Autodesk Inventor part; units mm, degrees
(part 4 of 4)
sketch "Эскиз10" plane through (23.5, 10.85, -93.6349) normal (0, 0, 1) x (1, 0, 0)
  arc A0 (0, 0) -> (-2.0546, 2.8471) centre (-3, 0) ccw projected
  line L0 (-2.0546, -10.85) -> (-2.0546, 2.8471) construction
  line L1 (0, -10.85) -> (-2.0546, -10.85) construction
  line L2 (0, -10.85) -> (0, 0) construction
  spline S0 degree 4 poles (-4.4081, 2.9941) (-4.3815, 2.997) (-4.3546, 2.999) (-4.3274, 3) (-4.3, 3) knots 0 0 0 0 0 1 1 1 1 1 projected
  line L3 (-4.4081, -1.0919) -> (-4.4081, 2.9941) construction
  line L4 (-3.5, -2) -> (-4.4081, -1.0919) projected
  line L5 (-3.5, -7) -> (-3.5, -2) construction
  line L6 (-4.4081, -7) -> (-3.5, -7) construction
  line L7 (-4.4081, -10.85) -> (-4.4081, -7) construction
  line L8 (-2.0546, -10.85) -> (-4.4081, -10.85) construction
  line L9 (-2.0546, -10.85) -> (-2.0546, 2.8471) construction
  spline S1 degree 6 poles (-3, 3) (-2.9139, 3) (-2.8267, 2.997) (-2.7386, 2.991) (-2.6499, 2.9817) (-2.5611, 2.9691) (-2.4019, 2.9407) (-2.3314, 2.926) (-2.2612, 2.9092) (-2.1915, 2.8904) (-2.1226, 2.8697) (-2.0546, 2.8471) knots 0 0 0 0 0 0 0 0.556009 0.556009 0.556009 0.556009 0.556009 1 1 1 1 1 1 1 projected
  line L10 (-4.3, 3) -> (-3, 3) projected
  arc A1 (-4.4081, 2.9941) -> (-5.3, 2) centre (-4.3, 2) ccw projected
  line L11 (-5.3, -0.2) -> (-5.3, 2) projected
  line L12 (-4.4081, -1.0919) -> (-5.3, -0.2) projected
  line L13 (-4.4081, -1.0919) -> (-4.4081, 2.9941) construction
  line L14 (-42.5919, -1.0919) -> (-42.5919, 2.9941) projected
  arc A2 (-41.7, 2) -> (-42.5919, 2.9941) centre (-42.7, 2) ccw projected
  line L15 (-42.5919, -1.0919) -> (-42.5919, 2.9941) projected
  line L16 (-41.7, -0.2) -> (-42.5919, -1.0919) projected
  line L17 (-41.7, -0.2) -> (-41.7, 2) projected
  spline S2 degree 7 poles (-42.7, 3) (-42.6843, 3) (-42.6687, 2.9997) (-42.6532, 2.9991) (-42.6378, 2.9983) (-42.6224, 2.9972) (-42.6071, 2.9958) (-42.5919, 2.9941) knots 0 0 0 0 0 0 0 0 1 1 1 1 1 1 1 1 projected
  line L18 (-44, 3) -> (-42.7, 3) projected
  spline S3 degree 5 poles (-44.9454, 2.8471) (-44.8643, 2.8741) (-44.782, 2.8982) (-44.6986, 2.9194) (-44.6145, 2.9376) (-44.4235, 2.9719) (-44.3163, 2.9862) (-44.2095, 2.9955) (-44.1039, 3) (-44, 3) knots 0 0 0 0 0 0 0.440959 0.440959 0.440959 0.440959 1 1 1 1 1 1 projected
  line L19 (-44.9454, -10.85) -> (-44.9454, 2.8471) construction
  line L20 (-42.5919, -10.85) -> (-44.9454, -10.85) construction
  line L21 (-42.5919, -10.85) -> (-42.5919, -7) construction
  line L22 (-43.5, -7) -> (-42.5919, -7) construction
  line L23 (-43.5, -7) -> (-43.5, -2) construction
  line L24 (-42.5919, -1.0919) -> (-43.5, -2) projected
  line L25 (-42.5919, -1.0919) -> (-42.5919, 2.9941) projected
  arc A3 (-44.9454, 2.8471) -> (-47, 0) centre (-44, 0) ccw projected
  line L26 (-47, -10.85) -> (-47, 0) construction
  line L27 (-44.9454, -10.85) -> (-47, -10.85) construction
  line L28 (-44.9454, -10.85) -> (-44.9454, 2.8471) construction
  line L29 (6.6851, -2.85) -> (-3.5, -2.85) construction
  line L30 (-3.0402, -2.85) -> (-3.5, -2.85) construction
  line L31 (0, -2.85) -> (-3.0402, -2.85) construction
  line L32 (0, -2.85) -> (1.5, -2.85) construction
  line L33 (1.5, -2.85) -> (3.522, -2.85) construction
  line L34 (3.522, -2.85) -> (6.6851, -2.85) construction
  line L35 (-43.5, -2.85) -> (-53.6851, -2.85) construction
  line L36 (-53.6851, -2.85) -> (-50.522, -2.85) construction
  line L37 (-50.522, -2.85) -> (-48.5, -2.85) construction
  line L38 (-48.5, -2.85) -> (-47, -2.85) construction
  line L39 (-43.9598, -2.85) -> (-47, -2.85) construction
  line L40 (-43.5, -2.85) -> (-43.9598, -2.85) construction
  line L41 (0, -10.85) -> (0, 0) projected
  line L42 (0, -2.85) -> (0, 0)
  line L43 (-3.5, -7) -> (-3.5, -2) projected
  line L44 (-3.5, -2.85) -> (-3.5, -2)
  line L45 (0, -2.85) -> (-3.5, -2.85)
  line L46 (-42.5919, -1.0919) -> (-43.5, -2) projected
  line L47 (-43.5, -2) -> (-43.5, -2.85)
  line L48 (-43.5, -7) -> (-43.5, -2) projected
  line L49 (-43.5, -2.85) -> (-47, -2.85)
  line L50 (-47, -10.85) -> (-47, 0) projected
  line L51 (-47, -2.85) -> (-47, 0)
  point P0 (-23.5, -10.85)
  point P1 (-44.9454, 2.8471)
  point P2 (-2.0546, 2.8471)
  constraints: 12 end point, 5 collinear, 1 perpendicular, 4 other
extrude "Выдавливание15" add sketch "Эскиз10" against normal blind 5.5
extrude "Выдавливание16" add sketch "Эскиз9" along normal up to surface (1.85 mm away) contours L103 A159 | A159 L103 A164 A165 A163 | A160 A161 L103 | L103 A162 A160 | A163 A165 A164 L106 L105 L104
fillet "Сопряжение3" radius 2 1 edges at (0, 2, -51)
sketch "Эскиз11" plane through (0, 0, 0) normal (0, -1, 0) x (1, 0, 0)
  circle A0 centre (0, -46) radius 1.6 projected
  circle A1 centre (24, -98.1071) radius 1.6 projected
  circle A2 centre (-24, -98.1071) radius 1.6 projected
  point P0 (0, 0)
extrude "Выдавливание17" cut sketch "Эскиз11" against normal up to surface (8 mm away)
sketch "Эскиз12" plane through (0, 36.5, 0) normal (0, 1, 0) x (1, 0, 0)
  arc A0 (46.0909, 86.4848) -> (42.0132, 88.5375) centre (0, 0) ccw
  line L0 (42.7346, 92.2321) -> (44.244, 93.7415) construction
  arc A1 (44.244, 93.7415) -> (43.9555, 95.3568) centre (43.5369, 94.4486) ccw construction
  arc A2 (43.9555, 95.3568) -> (21.2019, 102.8371) centre (0, 0) ccw construction
  arc A3 (21.2019, 102.8371) -> (20, 101.8577) centre (21, 101.8577) ccw construction
  line L1 (20, 101.8577) -> (20, 99) construction
  arc A4 (41.6155, 92.028) -> (20, 99) centre (0, 0) ccw construction
  arc A5 (41.6155, 92.028) -> (42.7346, 92.2321) centre (42.0275, 92.9392) ccw construction
  arc A6 (23.5, 96.5872) -> (25.5511, 97.7146) centre (24, 98.1071) ccw construction
  line L2 (23.5, 96.5872) -> (23.5, 92.2976) construction
  arc A7 (25, 94.2341) -> (23.5, 92.2976) centre (25.5, 92.2976) ccw construction
  arc A8 (25, 94.2341) -> (27.022, 95.4865) centre (24, 98.1071) ccw construction
  arc A9 (30.1851, 96.3839) -> (27.022, 95.4865) centre (29.2885, 93.521) ccw construction
  arc A10 (30.1851, 96.3839) -> (25.5511, 97.7146) centre (0, 0) ccw construction
  arc A11 (20.7476, 95.7786) -> (25, 94.2341) centre (24, 98.1071) ccw construction
  line L3 (20.5, 98.8977) -> (20.5, 47.4035) construction
  line L4 (21.4454, 47.6084) -> (23.5, 49.663) construction
  line L5 (23.5, 49.663) -> (23.5, 98.2281) construction
  arc A12 (-23.5, 96.5872) -> (-25.5511, 97.7146) centre (-24, 98.1071) ccw construction
  line L6 (-23.5, 98.2281) -> (-23.5, 49.663) construction
  line L7 (-23.5, 49.663) -> (-21.4454, 47.6084) construction
  line L8 (-20.5, 47.4035) -> (-20.5, 98.8977) construction
  arc A13 (-25.5511, 97.7146) -> (-23.5, 96.5872) centre (-24, 98.1071) ccw construction
  arc A14 (-25.5511, 97.7146) -> (-30.1851, 96.3839) centre (0, 0) ccw construction
  arc A15 (-27.022, 95.4865) -> (-30.1851, 96.3839) centre (-29.2885, 93.521) ccw construction
  arc A16 (-27.022, 95.4865) -> (-25, 94.2341) centre (-24, 98.1071) ccw construction
  arc A17 (-23.5, 92.2976) -> (-25, 94.2341) centre (-25.5, 92.2976) ccw construction
  line L9 (-23.5, 96.5872) -> (-23.5, 92.2976) construction
  arc A18 (-42.7346, 92.2321) -> (-41.6155, 92.028) centre (-42.0275, 92.9392) ccw construction
  arc A19 (-20, 99) -> (-41.6155, 92.028) centre (0, 0) ccw construction
  line L10 (-20, 99) -> (-20, 101.8577) construction
  arc A20 (-20, 101.8577) -> (-21.2019, 102.8371) centre (-21, 101.8577) ccw construction
  arc A21 (-21.2019, 102.8371) -> (-43.9555, 95.3568) centre (0, 0) ccw construction
  arc A22 (-43.9555, 95.3568) -> (-44.244, 93.7415) centre (-43.5369, 94.4486) ccw construction
  line L11 (-44.244, 93.7415) -> (-42.7346, 92.2321) construction
  arc A23 (-3.7645, 44.6477) -> (-5.2381, 46.3127) centre (-6.5878, 43.6335) ccw construction
  arc A24 (-6.2595, 46.1335) -> (-5.2381, 46.3127) centre (-6.2595, 49.1335) ccw construction
  line L12 (-6.2595, 46.1335) -> (-19.2746, 46.1335) construction
  arc A25 (-19.2746, 46.1335) -> (-21.6698, 47.1257) centre (-21.9203, 43.1335) ccw construction
  line L13 (-21.6698, 47.1257) -> (-42.4264, 67.8823) construction
  line L14 (-42.4264, 67.8823) -> (-34.2947, 76.014) construction
  arc A26 (-34.2947, 76.014) -> (-34.2947, 83.085) centre (-37.8302, 79.5495) ccw construction
  line L15 (-34.2947, 83.085) -> (-38.3892, 87.1795) construction
  arc A27 (-37.7453, 90.4395) -> (-38.3892, 87.1795) centre (-36.975, 88.5938) ccw construction
  arc A28 (-25.8102, 94.5401) -> (-37.7453, 90.4395) centre (0, 0) ccw construction
  arc A29 (-27.022, 95.4865) -> (-25.8102, 94.5401) centre (-24, 98.1071) ccw construction
  arc A30 (-27.022, 95.4865) -> (-30.1851, 96.3839) centre (-29.2885, 93.521) ccw construction
  arc A31 (-30.1851, 96.3839) -> (-41.6155, 92.028) centre (0, 0) ccw construction
  arc A32 (-42.7346, 92.2321) -> (-41.6155, 92.028) centre (-42.0275, 92.9392) ccw construction
  line L16 (-42.7346, 92.2321) -> (-44.244, 93.7415) construction
  arc A33 (-43.9555, 95.3568) -> (-44.244, 93.7415) centre (-43.5369, 94.4486) ccw construction
  arc A34 (-43.9555, 95.3568) -> (-48.6481, 93.0503) centre (0, 0) ccw projected
  arc A35 (-48.6481, 93.0503) -> (-49.3795, 88.2704) centre (-47.2582, 90.3917) ccw projected
  line L17 (-49.3795, 88.2704) -> (-46.3155, 85.2064) construction
  arc A36 (-46.3155, 73.8927) -> (-46.3155, 85.2064) centre (-51.9723, 79.5495) ccw construction
  line L18 (-46.3155, 73.8927) -> (-73.8927, 46.3155) construction
  arc A37 (-85.2064, 46.3155) -> (-73.8927, 46.3155) centre (-79.5495, 51.9723) ccw construction
  line L19 (-85.2064, 46.3155) -> (-88.2704, 49.3795) construction
  arc A38 (-88.2704, 49.3795) -> (-93.0503, 48.6481) centre (-90.3917, 47.2582) ccw construction
  arc A39 (-93.0503, 48.6481) -> (-93.0503, -48.6481) centre (0, 0) ccw construction
  arc A40 (-93.0503, -48.6481) -> (-88.2704, -49.3795) centre (-90.3917, -47.2582) ccw construction
  line L20 (-88.2704, -49.3795) -> (-85.2064, -46.3155) construction
  arc A41 (-73.8927, -46.3155) -> (-85.2064, -46.3155) centre (-79.5495, -51.9723) ccw construction
  line L21 (-73.8927, -46.3155) -> (-46.3155, -73.8927) construction
  arc A42 (-46.3155, -85.2064) -> (-46.3155, -73.8927) centre (-51.9723, -79.5495) ccw construction
  line L22 (-46.3155, -85.2064) -> (-49.3795, -88.2704) construction
  arc A43 (-49.3795, -88.2704) -> (-48.6481, -93.0503) centre (-47.2582, -90.3917) ccw construction
  arc A44 (-48.6481, -93.0503) -> (-45.42, -94.668) centre (0, 0) ccw construction
  arc A45 (-45.42, -94.668) -> (-43.0355, -94.1655) centre (-44.5548, -92.8648) ccw construction
  line L23 (-43.0355, -94.1655) -> (-18.3802, -65.3664) construction
  arc A46 (-17.477, -64.7643) -> (-18.3802, -65.3664) centre (-16.8609, -66.6671) ccw construction
  line L24 (-17.477, -64.7643) -> (-0.6161, -59.3045) construction
  arc A47 (0.6161, -59.3045) -> (-0.6161, -59.3045) centre (0, -61.2072) ccw construction
  line L25 (0.6161, -59.3045) -> (17.477, -64.7643) construction
  arc A48 (18.3802, -65.3664) -> (17.477, -64.7643) centre (16.8609, -66.6671) ccw construction
  line L26 (18.3802, -65.3664) -> (43.0355, -94.1655) construction
  arc A49 (43.0355, -94.1655) -> (45.42, -94.668) centre (44.5548, -92.8648) ccw construction
  arc A50 (45.42, -94.668) -> (48.6481, -93.0503) centre (0, 0) ccw construction
  arc A51 (48.6481, -93.0503) -> (49.3795, -88.2704) centre (47.2582, -90.3917) ccw construction
  line L27 (49.3795, -88.2704) -> (46.3155, -85.2064) construction
  arc A52 (46.3155, -73.8927) -> (46.3155, -85.2064) centre (51.9723, -79.5495) ccw construction
  line L28 (46.3155, -73.8927) -> (73.8927, -46.3155) construction
  arc A53 (85.2064, -46.3155) -> (73.8927, -46.3155) centre (79.5495, -51.9723) ccw construction
  line L29 (85.2064, -46.3155) -> (88.2704, -49.3795) construction
  arc A54 (88.2704, -49.3795) -> (93.0503, -48.6481) centre (90.3917, -47.2582) ccw construction
  arc A55 (93.0503, -48.6481) -> (93.0503, 48.6481) centre (0, 0) ccw construction
  arc A56 (93.0503, 48.6481) -> (88.2704, 49.3795) centre (90.3917, 47.2582) ccw construction
  line L30 (88.2704, 49.3795) -> (85.2064, 46.3155) construction
  arc A57 (73.8927, 46.3155) -> (85.2064, 46.3155) centre (79.5495, 51.9723) ccw construction
  line L31 (73.8927, 46.3155) -> (46.3155, 73.8927) construction
  arc A58 (46.3155, 85.2064) -> (46.3155, 73.8927) centre (51.9723, 79.5495) ccw construction
  line L32 (46.3155, 85.2064) -> (49.3795, 88.2704) construction
  arc A59 (49.3795, 88.2704) -> (48.6481, 93.0503) centre (47.2582, 90.3917) ccw projected
  arc A60 (48.6481, 93.0503) -> (43.9555, 95.3568) centre (0, 0) ccw construction
  arc A61 (44.244, 93.7415) -> (43.9555, 95.3568) centre (43.5369, 94.4486) ccw construction
  line L33 (44.244, 93.7415) -> (42.7346, 92.2321) construction
  arc A62 (41.6155, 92.028) -> (42.7346, 92.2321) centre (42.0275, 92.9392) ccw construction
  arc A63 (41.6155, 92.028) -> (30.1851, 96.3839) centre (0, 0) ccw construction
  arc A64 (30.1851, 96.3839) -> (27.022, 95.4865) centre (29.2885, 93.521) ccw construction
  arc A65 (25.8102, 94.5401) -> (27.022, 95.4865) centre (24, 98.1071) ccw construction
  arc A66 (37.7453, 90.4395) -> (25.8102, 94.5401) centre (0, 0) ccw construction
  arc A67 (38.3892, 87.1795) -> (37.7453, 90.4395) centre (36.975, 88.5938) ccw construction
  line L34 (38.3892, 87.1795) -> (34.2947, 83.085) construction
  arc A68 (34.2947, 83.085) -> (34.2947, 76.014) centre (37.8302, 79.5495) ccw construction
  line L35 (34.2947, 76.014) -> (42.4264, 67.8823) construction
  line L36 (42.4264, 67.8823) -> (21.6698, 47.1257) construction
  arc A69 (21.6698, 47.1257) -> (19.2746, 46.1335) centre (21.9203, 43.1335) ccw construction
  line L37 (19.2746, 46.1335) -> (6.2595, 46.1335) construction
  arc A70 (5.2381, 46.3127) -> (6.2595, 46.1335) centre (6.2595, 49.1335) ccw construction
  arc A71 (5.2381, 46.3127) -> (3.7645, 44.6477) centre (6.5878, 43.6335) ccw construction
  arc A72 (-3.7645, 44.6477) -> (3.7645, 44.6477) centre (0, 46) ccw construction
  line L38 (-19.2746, -46.1335) -> (19.2746, -46.1335) construction
  arc A73 (19.2746, -46.1335) -> (21.6698, -47.1257) centre (21.9203, -43.1335) ccw construction
  line L39 (21.6698, -47.1257) -> (42.4264, -67.8823) construction
  line L40 (42.4264, -67.8823) -> (37.1244, -73.1843) construction
  arc A74 (34.1909, -73.0707) -> (37.1244, -73.1843) centre (35.7102, -71.7701) ccw construction
  line L41 (34.1909, -73.0707) -> (25.4187, -62.8242) construction
  arc A75 (24.842, -61.8893) -> (25.4187, -62.8242) centre (28.1154, -60.5155) ccw construction
  line L42 (24.842, -61.8893) -> (23.8313, -59.4808) construction
  arc A76 (23.8313, -59.4808) -> (21.0049, -57.3328) centre (20.5578, -60.8546) ccw construction
  line L43 (21.0049, -57.3328) -> (15.1585, -56.5907) construction
  arc A77 (14.5119, -56.4463) -> (15.1585, -56.5907) centre (15.6055, -53.069) ccw construction
  line L44 (14.5119, -56.4463) -> (0.6161, -51.9466) construction
  arc A78 (0.6161, -51.9466) -> (-0.6161, -51.9466) centre (0, -53.8493) ccw construction
  line L45 (-0.6161, -51.9466) -> (-14.5119, -56.4463) construction
  arc A79 (-15.1585, -56.5907) -> (-14.5119, -56.4463) centre (-15.6055, -53.069) ccw construction
  line L46 (-15.1585, -56.5907) -> (-21.0049, -57.3328) construction
  arc A80 (-21.0049, -57.3328) -> (-23.8313, -59.4808) centre (-20.5578, -60.8546) ccw construction
  line L47 (-23.8313, -59.4808) -> (-24.842, -61.8893) construction
  arc A81 (-25.4187, -62.8242) -> (-24.842, -61.8893) centre (-28.1154, -60.5155) ccw construction
  line L48 (-25.4187, -62.8242) -> (-34.1909, -73.0707) construction
  arc A82 (-37.1244, -73.1843) -> (-34.1909, -73.0707) centre (-35.7102, -71.7701) ccw construction
  line L49 (-37.1244, -73.1843) -> (-42.4264, -67.8823) construction
  line L50 (-42.4264, -67.8823) -> (-21.6698, -47.1257) construction
  arc A83 (-21.6698, -47.1257) -> (-19.2746, -46.1335) centre (-21.9203, -43.1335) ccw construction
  circle A84 centre (0, -40) radius 1.6 construction
  arc A85 (3.6492, -38.362) -> (-3.6492, -38.362) centre (0, -40) ccw construction
  arc A86 (-6.3862, -40.1335) -> (-3.6492, -38.362) centre (-6.3862, -37.1335) ccw construction
  line L51 (-6.3862, -40.1335) -> (-19.2746, -40.1335) construction
  arc A87 (-19.2746, -40.1335) -> (-21.6698, -39.1414) centre (-21.9203, -43.1335) ccw construction
  line L52 (-21.6698, -39.1414) -> (-39.1414, -21.6698) construction
  arc A88 (-39.1414, -21.6698) -> (-40.1335, -19.2746) centre (-43.1335, -21.9203) ccw construction
  line L53 (-40.1335, -19.2746) -> (-40.1335, 19.2746) construction
  arc A89 (-40.1335, 19.2746) -> (-39.1414, 21.6698) centre (-43.1335, 21.9203) ccw construction
  line L54 (-39.1414, 21.6698) -> (-21.6698, 39.1414) construction
  arc A90 (-21.6698, 39.1414) -> (-19.2746, 40.1335) centre (-21.9203, 43.1335) ccw construction
  line L55 (-19.2746, 40.1335) -> (19.2746, 40.1335) construction
  arc A91 (19.2746, 40.1335) -> (21.6698, 39.1414) centre (21.9203, 43.1335) ccw construction
  line L56 (21.6698, 39.1414) -> (39.1414, 21.6698) construction
  arc A92 (39.1414, 21.6698) -> (40.1335, 19.2746) centre (43.1335, 21.9203) ccw construction
  line L57 (40.1335, 19.2746) -> (40.1335, -19.2746) construction
  arc A93 (40.1335, -19.2746) -> (39.1414, -21.6698) centre (43.1335, -21.9203) ccw construction
  line L58 (39.1414, -21.6698) -> (21.6698, -39.1414) construction
  arc A94 (21.6698, -39.1414) -> (19.2746, -40.1335) centre (21.9203, -43.1335) ccw construction
  line L59 (19.2746, -40.1335) -> (6.3862, -40.1335) construction
  arc A95 (3.6492, -38.362) -> (6.3862, -40.1335) centre (6.3862, -37.1335) ccw construction
  circle A96 centre (46, 0) radius 1.6 construction
  arc A97 (47.7906, -3.5768) -> (46.1335, -6.2595) centre (49.1335, -6.2595) ccw construction
  arc A98 (47.7906, -3.5768) -> (47.7906, 3.5768) centre (46, 0) ccw construction
  arc A99 (46.1335, 6.2595) -> (47.7906, 3.5768) centre (49.1335, 6.2595) ccw construction
  line L60 (46.1335, 6.2595) -> (46.1335, 19.2746) construction
  arc A100 (46.1335, 19.2746) -> (47.1257, 21.6698) centre (43.1335, 21.9203) ccw construction
  line L61 (47.1257, 21.6698) -> (67.8823, 42.4264) construction
  line L62 (67.8823, 42.4264) -> (76.014, 34.2947) construction
  arc A101 (76.014, 34.2947) -> (83.085, 34.2947) centre (79.5495, 37.8302) ccw construction
  line L63 (83.085, 34.2947) -> (87.1795, 38.3892) construction
  arc A102 (90.4395, 37.7453) -> (87.1795, 38.3892) centre (88.5938, 36.975) ccw construction
  arc A103 (97.9653, 2.6059) -> (90.4395, 37.7453) centre (0, 0) ccw construction
  arc A104 (97.9653, 2.6059) -> (97.9653, -2.6059) centre (101, 0) ccw construction
  arc A105 (90.4395, -37.7453) -> (97.9653, -2.6059) centre (0, 0) ccw construction
  arc A106 (87.1795, -38.3892) -> (90.4395, -37.7453) centre (88.5938, -36.975) ccw construction
  line L64 (87.1795, -38.3892) -> (83.085, -34.2947) construction
  arc A107 (83.085, -34.2947) -> (76.014, -34.2947) centre (79.5495, -37.8302) ccw construction
  line L65 (76.014, -34.2947) -> (67.8823, -42.4264) construction
  line L66 (67.8823, -42.4264) -> (47.1257, -21.6698) construction
  arc A108 (47.1257, -21.6698) -> (46.1335, -19.2746) centre (43.1335, -21.9203) ccw construction
  line L67 (46.1335, -19.2746) -> (46.1335, -6.2595) construction
  circle A109 centre (101, 0) radius 1.6 construction
  circle A110 centre (45.1111, -90.3659) radius 1.6 construction
  circle A111 centre (45.1111, 90.3659) radius 1.6 projected
  circle A112 centre (90.3659, 45.1111) radius 1.6 construction
  circle A113 centre (90.3659, -45.1111) radius 1.6 construction
  line L68 (63.6396, 46.669) -> (43.8406, 26.8701) construction
  arc A114 (41.0122, 26.8701) -> (43.8406, 26.8701) centre (42.4264, 28.2843) ccw construction
  line L69 (41.0122, 26.8701) -> (26.8701, 41.0122) construction
  arc A115 (26.8701, 43.8406) -> (26.8701, 41.0122) centre (28.2843, 42.4264) ccw construction
  line L70 (26.8701, 43.8406) -> (46.669, 63.6396) construction
  line L71 (46.669, 63.6396) -> (63.6396, 46.669) construction
  circle A116 centre (43.1335, 21.9203) radius 1.6 construction
  circle A117 centre (21.9203, -43.1335) radius 1.6 construction
  circle A118 centre (43.1335, -21.9203) radius 1.6 construction
  circle A119 centre (21.9203, 43.1335) radius 1.6 construction
  circle A120 centre (79.5495, -37.8302) radius 1.6 construction
  circle A121 centre (37.8302, 79.5495) radius 1.6 construction
  circle A122 centre (79.5495, 37.8302) radius 1.6 construction
  circle A123 centre (20.5578, -60.8546) radius 1.55 construction
  circle A124 centre (37.8302, -79.5495) radius 1.6 construction
  line L72 (46.669, -63.6396) -> (26.8701, -43.8406) construction
  arc A125 (26.8701, -41.0122) -> (26.8701, -43.8406) centre (28.2843, -42.4264) ccw construction
  line L73 (26.8701, -41.0122) -> (41.0122, -26.8701) construction
  arc A126 (43.8406, -26.8701) -> (41.0122, -26.8701) centre (42.4264, -28.2843) ccw construction
  line L74 (43.8406, -26.8701) -> (63.6396, -46.669) construction
  line L75 (63.6396, -46.669) -> (46.669, -63.6396) construction
  circle A127 centre (-46, 0) radius 1.6 construction
  circle A128 centre (-101, 0) radius 1.6 construction
  arc A129 (-47.7906, 3.5768) -> (-46.1335, 6.2595) centre (-49.1335, 6.2595) ccw construction
  arc A130 (-47.7906, 3.5768) -> (-47.7906, -3.5768) centre (-46, 0) ccw construction
  arc A131 (-46.1335, -6.2595) -> (-47.7906, -3.5768) centre (-49.1335, -6.2595) ccw construction
  line L76 (-46.1335, -6.2595) -> (-46.1335, -19.2746) construction
  arc A132 (-46.1335, -19.2746) -> (-47.1257, -21.6698) centre (-43.1335, -21.9203) ccw construction
  line L77 (-47.1257, -21.6698) -> (-67.8823, -42.4264) construction
  line L78 (-67.8823, -42.4264) -> (-76.014, -34.2947) construction
  arc A133 (-76.014, -34.2947) -> (-83.085, -34.2947) centre (-79.5495, -37.8302) ccw construction
  line L79 (-83.085, -34.2947) -> (-87.1795, -38.3892) construction
  arc A134 (-90.4395, -37.7453) -> (-87.1795, -38.3892) centre (-88.5938, -36.975) ccw construction
  arc A135 (-97.9653, -2.6059) -> (-90.4395, -37.7453) centre (0, 0) ccw construction
  arc A136 (-97.9653, -2.6059) -> (-97.9653, 2.6059) centre (-101, 0) ccw construction
  arc A137 (-90.4395, 37.7453) -> (-97.9653, 2.6059) centre (0, 0) ccw construction
  arc A138 (-87.1795, 38.3892) -> (-90.4395, 37.7453) centre (-88.5938, 36.975) ccw construction
  line L80 (-87.1795, 38.3892) -> (-83.085, 34.2947) construction
  arc A139 (-83.085, 34.2947) -> (-76.014, 34.2947) centre (-79.5495, 37.8302) ccw construction
  line L81 (-76.014, 34.2947) -> (-67.8823, 42.4264) construction
  line L82 (-67.8823, 42.4264) -> (-47.1257, 21.6698) construction
  arc A140 (-47.1257, 21.6698) -> (-46.1335, 19.2746) centre (-43.1335, 21.9203) ccw construction
  line L83 (-46.1335, 19.2746) -> (-46.1335, 6.2595) construction
  circle A141 centre (-45.1111, -90.3659) radius 1.6 construction
  circle A142 centre (-45.1111, 90.3659) radius 1.6 projected
  circle A143 centre (-90.3659, 45.1111) radius 1.6 construction
  circle A144 centre (-90.3659, -45.1111) radius 1.6 construction
  line L84 (-46.669, 63.6396) -> (-26.8701, 43.8406) construction
  arc A145 (-26.8701, 41.0122) -> (-26.8701, 43.8406) centre (-28.2843, 42.4264) ccw construction
  line L85 (-26.8701, 41.0122) -> (-41.0122, 26.8701) construction
  arc A146 (-43.8406, 26.8701) -> (-41.0122, 26.8701) centre (-42.4264, 28.2843) ccw construction
  line L86 (-43.8406, 26.8701) -> (-63.6396, 46.669) construction
  line L87 (-63.6396, 46.669) -> (-46.669, 63.6396) construction
  line L88 (-63.6396, -46.669) -> (-43.8406, -26.8701) construction
  arc A147 (-41.0122, -26.8701) -> (-43.8406, -26.8701) centre (-42.4264, -28.2843) ccw construction
  line L89 (-41.0122, -26.8701) -> (-26.8701, -41.0122) construction
  arc A148 (-26.8701, -43.8406) -> (-26.8701, -41.0122) centre (-28.2843, -42.4264) ccw construction
  line L90 (-26.8701, -43.8406) -> (-46.669, -63.6396) construction
  line L91 (-46.669, -63.6396) -> (-63.6396, -46.669) construction
  circle A149 centre (-21.9203, -43.1335) radius 1.6 construction
  circle A150 centre (-43.1335, -21.9203) radius 1.6 construction
  circle A151 centre (-43.1335, 21.9203) radius 1.6 construction
  circle A152 centre (-21.9203, 43.1335) radius 1.6 construction
  circle A153 centre (-37.8302, 79.5495) radius 1.6 construction
  circle A154 centre (-79.5495, 37.8302) radius 1.6 construction
  circle A155 centre (-79.5495, -37.8302) radius 1.6 construction
  circle A156 centre (-20.5578, -60.8546) radius 1.55 construction
  circle A157 centre (-37.8302, -79.5495) radius 1.6 construction
  arc A158 (41.4241, 88.8147) -> (41.4975, 92.0812) centre (45.1111, 90.3659) ccw construction
  arc A159 (41.6155, 92.028) -> (20, 99) centre (0, 0) ccw projected
  arc A160 (41.6155, 92.028) -> (41.4975, 92.0812) centre (0, 0) ccw construction
  arc A161 (41.1291, 90.7454) -> (41.1834, 89.6088) centre (45.1111, 90.3659) ccw
  arc A162 (39.9288, 92.7723) -> (20, 99) centre (0, 0) ccw construction
  arc A163 (41.1291, 90.7454) -> (39.9288, 92.7723) centre (39.1381, 90.9352) ccw
  arc A164 (85.9577, 47.0668) -> (47.0668, 85.9577) centre (0, 0) ccw construction
  arc A165 (41.4241, 88.8147) -> (85.9577, 47.0668) centre (0, 0) ccw construction
  arc A166 (41.1834, 89.6088) -> (42.0132, 88.5375) centre (42.6562, 89.8927) ccw
  line L92 (46.3155, 85.2064) -> (49.3795, 88.2704) construction
  line L93 (49.3795, 88.2704) -> (47.8571, 86.7479)
  arc A167 (46.0909, 86.4848) -> (47.8571, 86.7479) centre (46.7964, 87.8086) ccw
  arc A168 (48.6481, 93.0503) -> (43.9555, 95.3568) centre (0, 0) ccw projected
  arc A169 (48.6481, 93.0503) -> (43.9555, 95.3568) centre (0, 0) ccw
  line L94 (43.9555, 95.3568) -> (39.9288, 92.7723)
  line L95 (2.9667, 52.9944) -> (-2.9667, 52.9944) construction
  line L96 (2.9667, 52.9944) -> (2.9667, 97.4549) construction
  arc A170 (2.9667, 97.4549) -> (-2.9667, 97.4549) centre (0, 0) ccw construction
  line L97 (-2.9667, 97.4549) -> (-2.9667, 52.9944) construction
  line L98 (0, 46) -> (0, 97.5) construction
  arc A171 (20.4598, 95.3292) -> (-20.4598, 95.3292) centre (0, 0) ccw construction
  arc A172 (49.3795, 88.2704) -> (48.6481, 93.0503) centre (47.2582, 90.3917) ccw
  line L99 (-43.9555, 95.3568) -> (-39.9288, 92.7723)
  arc A173 (-41.1834, 89.6088) -> (-41.1291, 90.7454) centre (-45.1111, 90.3659) ccw
  arc A174 (-39.9288, 92.7723) -> (-41.1291, 90.7454) centre (-39.1381, 90.9352) ccw
  arc A175 (-42.0132, 88.5375) -> (-41.1834, 89.6088) centre (-42.6562, 89.8927) ccw
  arc A176 (-42.0132, 88.5375) -> (-46.0909, 86.4848) centre (0, 0) ccw
  line L100 (-49.3795, 88.2704) -> (-47.8571, 86.7479)
  arc A177 (-47.8571, 86.7479) -> (-46.0909, 86.4848) centre (-46.7964, 87.8086) ccw
  arc A178 (-43.9555, 95.3568) -> (-48.6481, 93.0503) centre (0, 0) ccw construction
  arc A179 (-43.9555, 95.3568) -> (-48.6481, 93.0503) centre (0, 0) ccw construction
  dimension "d170" = 196
  dimension "d171" = 8
  dimension "d172" = 2
  dimension "d173" = 1.5
  dimension "d174" = 1.5
  dimension "d175" = 105
  constraints: 44 point on circle, 18 centre point, 11 symmetric about line, 10 end point, 8 tangent, 3 point on line, 2 coincident, 1 collinear, 9 other
  measures "d170" diameter of A0
  measures "d171" diameter of A158
  measures "d172" radius of A163
  measures "d173" radius of A166
  measures "d174" radius of A167
  measures "d175" radius of A169
extrude "Выдавливание18" add sketch "Эскиз12" against normal blind 35
